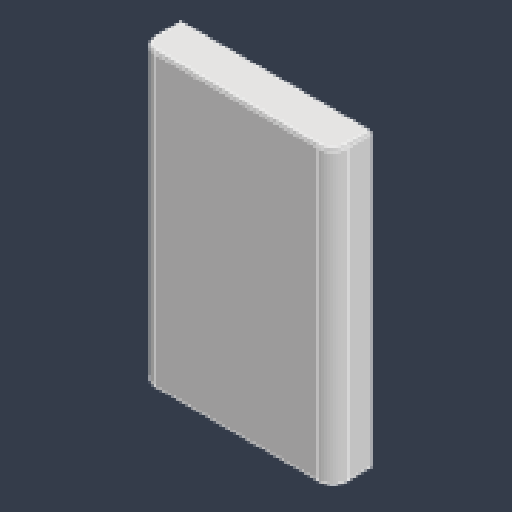
# Autodesk Inventor part: Battery
Saved by Autodesk Inventor 2023.4 (Build 274418000, 418)
## iProperties
Created: 2024-02-28
Part Number: Battery
Material: Generic
Document SubType Name: Modeling
Designer: JoaoSilva
Density: 1 g/cm^3
Appearance: Default
Author: JoaoSilva
Autodesk Inventor part; units mm, degrees
ref_plane "YZ Plane" through (0, 0, 0) normal (1, 0, 0) x (0, 1, 0)
ref_plane "XZ Plane" through (0, 0, 0) normal (0, 1, 0) x (-1, 0, 0)
ref_plane "XY Plane" through (0, 0, 0) normal (0, 0, 1) x (1, 0, 0)
sketch "Sketch1" plane through (0, 0, 0) normal (0, 0, 1) x (1, 0, 0)
  line L0 (-19.9, 30.25) -> (19.9, 30.25)
  line L1 (19.9, 30.25) -> (19.9, -30.25)
  line L2 (19.9, -30.25) -> (-19.9, -30.25)
  line L3 (-19.9, -30.25) -> (-19.9, 30.25)
  line L4 (-19.9, 30.25) -> (19.9, -30.25) construction
  line L5 (19.9, 30.25) -> (-19.9, -30.25) construction
  point P0 (0, 0)
  dimension "d0" = 39.8
  dimension "d1" = 60.5
  constraints: 12 end point, 2 midpoint, 2 parallel, 1 horizontal, 1 perpendicular
  measures "d0" distance of L1.end L2.end
  measures "d1" distance of L0.end L1.end
extrude "Extrusion1" add sketch "Sketch1" along normal mid plane 8
fillet "Fillet1" radius 3 2 edges at (19.9, 0, 4) (-19.9, 0, 4)
fillet "Fillet2" radius 0.5 10 edges at (-19.0213, 30.25, 3.1213) (-19.9, 30.25, -1.5) (19.0213, 30.25, 3.1213) (19.9, 30.25, -1.5) (0, 30.25, 4) (19.0213, -30.25, 3.1213) (19.9, -30.25, -1.5) (-19.0213, -30.25, 3.1213) (-19.9, -30.25, -1.5) (0, -30.25, 4)
body "Solid1"
